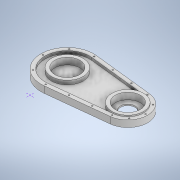
# Autodesk Inventor part: Klapp_Hinten_Abdeckung
Saved by Autodesk Inventor 2021 (Build 250183000, 183)
## iProperties
Created: 2021-01-19
Part Number: Klapp_Hinten_Abdeckung
Material: Generisch
Document SubType Name: Modeling
Designer: Jaro Machnow
Density: 1 g/cm^3
Appearance: Vorgabe
Author: Jaro Machnow
Autodesk Inventor part; units mm, degrees
ref_plane "YZ Plane" through (0, 0, 0) normal (1, 0, 0) x (0, 1, 0)
ref_plane "XZ Plane" through (0, 0, 0) normal (0, 1, 0) x (-1, 0, 0)
ref_plane "XY Plane" through (0, 0, 0) normal (0, 0, 1) x (1, 0, 0)
sketch "Skizze7" plane through (0, 0, 0) normal (0, -1, 0) x (1, 0, 0)
  point P0 (-1.8443, 26.478)
sketch "Skizze1" plane through (0, 0, 0) normal (0, 1, 0) x (-1, 0, 0)
  arc A0 (-2.1739, -19.8815) -> (-2.1739, 19.8815) centre (0, 0) ccw
  arc A1 (-47.6304, 14.9111) -> (-47.6304, -14.9111) centre (-46, 0) ccw
  line L0 (-2.1739, 19.8815) -> (-47.6304, 14.9111)
  line L1 (-2.1739, -19.8815) -> (-47.6304, -14.9111)
  line L2 (45.0235, 0) -> (-115.148, 0) construction
  dimension "d0" = 40
  dimension "d1" = 30
  dimension "d2" = 46
  constraints: 6 end point, 4 point on circle, 4 tangent, 2 centre point, 2 horizontal, 1 coincident, 1 point on line
  measures "d0" diameter of A0
  measures "d1" diameter of A1
  measures "d2" distance of A1.centre point (0, 0)
extrude "Extrusion1" add sketch "Skizze1" along normal blind 5
shell "Wandung1" thickness 3 removed faces 1 at (17.3261, 5, -4.9704)
sketch "Skizze2" plane through (0, 3, 0) normal (0, 1, 0) x (1, 0, 0)
  circle A0 centre (0, 0) radius 9.5
  circle A1 centre (0, 0) radius 12
  dimension "d6" = 19
  dimension "d7" = 24
  constraints: 2 centre point, 2 coincident
  measures "d6" diameter of A0
  measures "d7" diameter of A1
extrude "Extrusion2" add sketch "Skizze2" along normal blind 3
sketch "Skizze3" plane through (0, 3, 0) normal (0, 1, 0) x (1, 0, 0)
  arc A0 (47.3043, -11.9289) -> (47.3043, 11.9289) centre (46, 0) ccw projected
  circle A1 centre (46, 0) radius 9.5
  circle A2 centre (46, 0) radius 12
  point P0 (0, 0)
  point P1 (47.3043, -11.9289)
  dimension "d10" = 19
  constraints: 2 centre point, 2 coincident
  measures "d10" diameter of A1
extrude "Extrusion3" add sketch "Skizze3" along normal blind 3
sketch "Skizze4" plane through (0, 3, 0) normal (0, 1, 0) x (1, 0, 0)
  circle A0 centre (0, 0) radius 9.5
  constraints: 1 centre point, 1 coincident
extrude "Extrusion4" cut sketch "Skizze4" against normal blind 2
sketch "Skizze5" plane through (46, 3, 0) normal (0, 1, 0) x (1, 0, 0)
  circle A0 centre (0, 0) radius 9.5
  point P0 (-46, 0)
  constraints: 1 centre point
extrude "Extrusion5" cut sketch "Skizze5" against normal blind 2
sketch "Skizze6" plane through (46, 1, 0) normal (0, 1, 0) x (1, 0, 0)
  point P0 (-46, 0)
  point P1 (0, 0)
  point P2 (0, 0)
  constraints: 1 coincident
hole "Bohrung1" at (46, 1, 0) direction (0, -1, 0) diameter 11 end through all
sketch "Skizze8" plane through (0, 5, 0) normal (0, 1, 0) x (1, 0, 0)
  arc A0 (1.8478, 16.8993) -> (1.8478, -16.8993) centre (0, 0) ccw projected
  arc A1 (2.1739, 19.8815) -> (2.1739, -19.8815) centre (0, 0) ccw projected
  line L0 (47.3043, -11.9289) -> (1.8478, -16.8993) projected
  line L1 (2.1739, -19.8815) -> (47.6304, -14.9111) projected
  arc A2 (47.6304, -14.9111) -> (47.6304, 14.9111) centre (46, 0) ccw projected
  circle A3 centre (46, 0) radius 12 projected
  line L2 (1.8478, 16.8993) -> (47.3043, 11.9289) projected
  line L3 (47.6304, 14.9111) -> (2.1739, 19.8815) projected
  arc A4 (2.0109, 18.3904) -> (2.0109, -18.3904) centre (0, 0) ccw
  line L4 (2.0109, 18.3904) -> (47.4674, 13.42)
  arc A5 (47.4674, -13.42) -> (47.4674, 13.42) centre (46, 0) ccw
  line L5 (47.4674, -13.42) -> (2.0109, -18.3904)
  line L6 (47.4674, 13.42) -> (46, 0) construction
  line L7 (46, 0) -> (47.4674, -13.42) construction
  line L8 (0, 0) -> (2.0109, -18.3904) construction
  line L9 (0, 0) -> (2.0109, 18.3904) construction
  point P0 (0, -18.5)
  point P1 (56.0514, -9.0122)
  point P2 (59.5, 0)
  point P3 (56.0513, 9.0123)
  point P4 (47.4673, 13.42)
  point P5 (-12.3501, -13.7741)
  point P6 (-18.5, 0)
  point P7 (-12.3501, 13.774)
  point P8 (2.0108, 18.3904)
  point P9 (17.9161, -16.6513)
  point P10 (33.8213, -14.9121)
  point P11 (17.9161, 16.6513)
  point P12 (17.916, 16.6513)
  point P13 (33.8213, 14.9121)
  point P14 (33.8212, 14.9121)
  dimension "d24" = 1.5
  dimension "d26" = 167.52
  dimension "d29" = 167.52
  dimension "d31" = 167.52
  dimension "d34" = 192.48
  dimension "d38" = 16
  dimension "d45" = 16
  constraints: 12 end point, 6 point on circle, 2 centre point, 1 coincident, 21 other
  measures "d24" radial gap between concentric circles of A1 A4
  measures "d26" angle of L7 L6
  measures "d31" angle of L9 L8
  measures "d38" distance of point (2.011, -18.39) point (17.916, -16.651)
  measures "d45" distance of L4.start point (17.916, 16.651)
hole "Bohrung2" at (2.0109, 5, 18.3904) at (-12.3501, 5, 13.7741) at (-18.5, 5, 0) at (-12.3501, 5, -13.774) at (2.0108, 5, -18.3904) at (17.916, 5, -16.6513) at (33.8213, 5, -14.9121) at (47.4673, 5, -13.42) at (56.0513, 5, -9.0123) at (59.5, 5, 0) at (56.0514, 5, 9.0122) at (47.4674, 5, 13.42) at (33.8213, 5, 14.9121) at (17.9161, 5, 16.6513) direction (0, -1, 0) diameter 1 end through all
